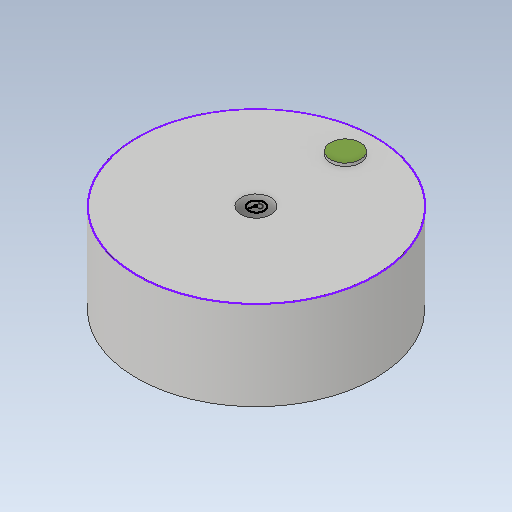
# Autodesk Inventor part: Part1
Saved by Autodesk Inventor 2020.2 (Build 242310000, 310)
## iProperties
Created: 2020-03-02
Part Number: Part1
Material: Generic
Document SubType Name: Modeling
Designer: Hp
Density: 1 g/cm^3
Appearance: Default
Author: Hp
Autodesk Inventor part; units mm, degrees
ref_plane "YZ Plane" through (0, 0, 0) normal (1, 0, 0) x (0, 1, 0)
ref_plane "XZ Plane" through (0, 0, 0) normal (0, 1, 0) x (-1, 0, 0)
ref_plane "XY Plane" through (0, 0, 0) normal (0, 0, 1) x (1, 0, 0)
sketch "Sketch1" plane through (0, 0, 0) normal (0, 1, 0) x (-1, 0, 0)
  circle A0 centre (0, 0) radius 20
  dimension "d24" = 40
  constraints: 1 centre point
  measures "d24" diameter of A0
extrude "Extrusion1" add sketch "Sketch1" along normal blind 50
sketch "Sketch2" plane through (0, 50, 0) normal (0, 1, 0) x (1, 0, 0)
  circle A0 centre (0, 0) radius 55
  dimension "d3" = 110
  constraints: 1 centre point, 1 coincident
  measures "d3" diameter of A0
extrude "Extrusion2" add sketch "Sketch2" against normal blind 50
sketch "Sketch3" plane through (0, 50, 0) normal (0, 1, 0) x (1, 0, 0)
  circle A0 centre (0, 0) radius 5
  dimension "d6" = 10
  constraints: 1 centre point, 1 coincident
  measures "d6" diameter of A0
extrude "Extrusion3" cut sketch "Sketch3" against normal blind 50
sketch "Sketch4" plane through (0, 50, 0) normal (0, 1, 0) x (1, 0, 0)
  circle A0 centre (0, -45) radius 5
  point P0 (0, 0)
  dimension "d9" = 10
  constraints: 1 centre point
  measures "d9" diameter of A0
extrude "Extrusion4" add sketch "Sketch4" along normal blind 1
sketch "Sketch5" plane through (0, 50, 0) normal (0, 1, 0) x (1, 0, 0)
  circle A0 centre (0, 0) radius 40
  dimension "d12" = 80
  constraints: 1 centre point, 1 coincident
  measures "d12" diameter of A0
extrude "Extrusion5" cut sketch "Sketch5" against normal through all keep common part
sketch "Sketch6" plane through (0, 50, 0) normal (0, 1, 0) x (1, 0, 0)
  circle A0 centre (0, 0) radius 40
  constraints: 1 centre point, 1 coincident
sketch "Sketch7" plane through (0, 0, 0) normal (0, -1, 0) x (1, 0, 0)
  circle A0 centre (0, 0) radius 40
  constraints: 1 centre point, 1 coincident
extrude "Extrusion6" cut sketch "Sketch7" against normal blind 10
sketch "Sketch8" plane through (0, 50, 0) normal (0, 1, 0) x (1, 0, 0)
  circle A0 centre (0, 30) radius 5
  point P0 (0, 0)
  dimension "d17" = 10
  constraints: 1 centre point
  measures "d17" diameter of A0
extrude "Extrusion7" add sketch "Sketch8" along normal blind 1
sketch "Sketch9" plane through (0, 50, 0) normal (0, 1, 0) x (1, 0, 0)
  circle A0 centre (0, 0) radius 2.5
  dimension "d20" = 5
  constraints: 1 centre point, 1 coincident
  measures "d20" diameter of A0
sketch "Sketch10" plane through (0, 10, 0) normal (0, -1, 0) x (1, 0, 0)
  circle A0 centre (0, 0) radius 5 projected
  circle A1 centre (0, 0) radius 40
  constraints: 1 centre point, 1 coincident
extrude "Extrusion8" cut sketch "Sketch10" against normal blind 10
body "Solid1"
